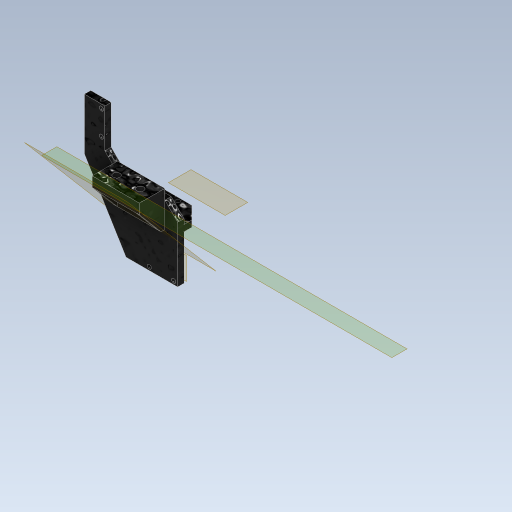
# Autodesk Inventor part: Suporte Switch Límite
Saved by Autodesk Inventor 2024.2 (Build 282272000, 272)
## iProperties
Created: 2024-01-17
Part Number: Suporte Switch Límite
Material: PET Plastic
Document SubType Name: Modeling
Designer: juanp
Density: 1.541 g/cm^3
Appearance: Black
Author: juanp
Autodesk Inventor part; units mm, degrees
ref_plane "YZ Plane" through (0, 0, 0) normal (1, 0, 0) x (0, 1, 0)
ref_plane "XZ Plane" through (0, 0, 0) normal (0, 1, 0) x (-1, 0, 0)
ref_plane "Work Plane1" through (0, 3, 3) normal (0, 0, 1) x (1, 0, 0)
sketch "Sketch1" plane through (0, 3, 3) normal (0, 0, 1) x (1, 0, 0)
  line L0 (-20.25, 5.05) -> (-20.25, -11.05) projected
  line L1 (-20.25, -11.05) -> (20.25, -11.05) projected
  line L2 (20.25, -11.05) -> (20.25, 5.05) projected
  line L3 (20.25, 5.05) -> (-20.25, 5.05) projected
  line L4 (-7.83, -4.67) -> (-7.83, -4.03) construction
  line L5 (-8.47, -4.67) -> (-7.83, -4.67) construction
  line L6 (-8.47, -4.03) -> (-8.47, -4.67) construction
  line L7 (-7.83, -4.03) -> (-8.47, -4.03) construction
  line L8 (-7.83, -7.17) -> (-7.83, -6.53) construction
  line L9 (-8.47, -7.17) -> (-7.83, -7.17) construction
  line L10 (-8.47, -6.53) -> (-8.47, -7.17) construction
  line L11 (-7.83, -6.53) -> (-8.47, -6.53) construction
  line L12 (2.725, -2.1031) -> (1.875, -2.1031) construction
  line L13 (2.725, -2.9531) -> (2.725, -2.1031) construction
  line L14 (1.875, -2.9531) -> (2.725, -2.9531) construction
  line L15 (1.875, -2.1031) -> (1.875, -2.9531) construction
  line L16 (7.875, -2.1031) -> (7.025, -2.1031) construction
  line L17 (7.875, -2.9531) -> (7.875, -2.1031) construction
  line L18 (7.025, -2.9531) -> (7.875, -2.9531) construction
  line L19 (7.025, -2.1031) -> (7.025, -2.9531) construction
  line L20 (13.025, -2.1031) -> (12.175, -2.1031) construction
  line L21 (13.025, -2.9531) -> (13.025, -2.1031) construction
  line L22 (12.175, -2.9531) -> (13.025, -2.9531) construction
  line L23 (12.175, -2.1031) -> (12.175, -2.9531) construction
  line L24 (-7.83, -2.17) -> (-7.83, -1.53) construction
  line L25 (-8.47, -2.17) -> (-7.83, -2.17) construction
  line L26 (-8.47, -1.53) -> (-8.47, -2.17) construction
  line L27 (-7.83, -1.53) -> (-8.47, -1.53) construction
  line L28 (-7.83, 0.33) -> (-7.83, 0.97) construction
  line L29 (-8.47, 0.33) -> (-7.83, 0.33) construction
  line L30 (-8.47, 0.97) -> (-8.47, 0.33) construction
  line L31 (-7.83, 0.97) -> (-8.47, 0.97) construction
  circle A0 centre (-16.75, 2.4) radius 1.5 construction
  circle A1 centre (17.15, -8.4) radius 1.5 construction
  circle A2 centre (-1.95, -8.4) radius 1.5 construction
  circle A3 centre (-16.75, -8.4) radius 1.5 construction
  line L32 (-53, 42.95) -> (-36.9, 42.95) projected
  line L33 (-36.9, 42.95) -> (-36.9, 83.45) projected
  line L34 (-36.9, 83.45) -> (-53, 83.45) projected
  line L35 (-53, 83.45) -> (-53, 42.95) projected
  line L36 (-43.28, 55.37) -> (-43.92, 55.37) construction
  line L37 (-43.28, 54.73) -> (-43.28, 55.37) construction
  line L38 (-43.92, 54.73) -> (-43.28, 54.73) construction
  line L39 (-43.92, 55.37) -> (-43.92, 54.73) construction
  line L40 (-40.78, 55.37) -> (-41.42, 55.37) construction
  line L41 (-40.78, 54.73) -> (-40.78, 55.37) construction
  line L42 (-41.42, 54.73) -> (-40.78, 54.73) construction
  line L43 (-41.42, 55.37) -> (-41.42, 54.73) construction
  line L44 (-45.8469, 65.925) -> (-45.8469, 65.075) construction
  line L45 (-44.9969, 65.925) -> (-45.8469, 65.925) construction
  line L46 (-44.9969, 65.075) -> (-44.9969, 65.925) construction
  line L47 (-45.8469, 65.075) -> (-44.9969, 65.075) construction
  line L48 (-45.8469, 71.075) -> (-45.8469, 70.225) construction
  line L49 (-44.9969, 71.075) -> (-45.8469, 71.075) construction
  line L50 (-44.9969, 70.225) -> (-44.9969, 71.075) construction
  line L51 (-45.8469, 70.225) -> (-44.9969, 70.225) construction
  line L52 (-45.8469, 76.225) -> (-45.8469, 75.375) construction
  line L53 (-44.9969, 76.225) -> (-45.8469, 76.225) construction
  line L54 (-44.9969, 75.375) -> (-44.9969, 76.225) construction
  line L55 (-45.8469, 75.375) -> (-44.9969, 75.375) construction
  line L56 (-45.78, 55.37) -> (-46.42, 55.37) construction
  line L57 (-45.78, 54.73) -> (-45.78, 55.37) construction
  line L58 (-46.42, 54.73) -> (-45.78, 54.73) construction
  line L59 (-46.42, 55.37) -> (-46.42, 54.73) construction
  line L60 (-48.28, 55.37) -> (-48.92, 55.37) construction
  line L61 (-48.28, 54.73) -> (-48.28, 55.37) construction
  line L62 (-48.92, 54.73) -> (-48.28, 54.73) construction
  line L63 (-48.92, 55.37) -> (-48.92, 54.73) construction
  circle A4 centre (-50.35, 46.45) radius 1.5 construction
  circle A5 centre (-39.55, 80.35) radius 1.5 construction
  circle A6 centre (-39.55, 61.25) radius 1.5 construction
  circle A7 centre (-39.55, 46.45) radius 1.5 construction
  circle A8 centre (-1.95, -8.4) radius 1.65
  circle A9 centre (17.15, -8.4) radius 1.65
  circle A10 centre (-39.55, 61.25) radius 1.65
  circle A11 centre (-39.55, 80.35) radius 1.65
  circle A12 centre (-1.95, -8.4) radius 2.65
  circle A13 centre (17.15, -8.4) radius 2.65
  circle A14 centre (-39.55, 61.25) radius 2.65
  circle A15 centre (-39.55, 80.35) radius 2.65
  line L64 (-20.25, 20.94) -> (20.25, 20.94) projected
  line L65 (-20.25, 20.94) -> (20.25, 20.94)
  line L66 (20.25, 20.94) -> (20.25, 28.94)
  line L67 (20.25, 28.94) -> (-20.25, 28.94)
  line L68 (-20.25, 28.94) -> (-20.25, 20.94)
  line L69 (-20.25, -11.05) -> (-53, 42.95)
  line L70 (20.25, 5.05) -> (20.25, 20.94)
  line L71 (20.25, 28.94) -> (20.25, 42.95)
  line L72 (20.25, 42.95) -> (-36.9, 42.95)
  line L73 (-25.9738, 88.007) -> (-9.8738, 88.007)
  line L74 (-9.8738, 88.007) -> (-9.8738, 47.507)
  line L75 (-9.8738, 47.507) -> (-25.9738, 47.507)
  line L76 (-25.9738, 47.507) -> (-25.9738, 88.007)
  line L77 (-12.5238, 84.907) -> (-12.5238, 65.807) construction
  circle A16 centre (-12.5238, 84.907) radius 1.5
  circle A17 centre (-12.5238, 65.807) radius 1.5
  point P0 (0, -3)
  dimension "d0" = 0.15
  dimension "d2" = 1
  dimension "d3" = 8
  dimension "d37" = 40.5
  dimension "d38" = 16.1
  dimension "d39" = 19.1
  dimension "d40" = 3
  dimension "d41" = 2.65
  dimension "d42" = 3.1
  dimension "d43" = 3
  dimension "d44" = 19.1
  dimension "d45" = 3.1
  dimension "d46" = 2.65
  dimension "d47" = 16.1
  dimension "d48" = 40.5
  constraints: 26 end point, 10 centre point, 7 equal radius, 4 parallel, 3 horizontal, 2 coincident, 2 perpendicular, 1 collinear, 1 point on line, 1 vertical
  measures "d0" radial gap between concentric circles of A2 A8
  measures "d2" radial gap between concentric circles of A12 A8
  measures "d3" distance between parallel lines of L67 L64
  measures "d37" distance of L32.end L33.end
  measures "d38" distance of L33.end L34.end
  measures "d39" distance of A5.centre A6.centre
  measures "d40" diameter of A5
  measures "d41" distance from line of L33 A5.centre
  measures "d42" distance from line of L34 A5.centre
  measures "d43" diameter of A16
  measures "d44" distance of L77.start L77.end
  measures "d45" distance from line of L73 L77.start
  measures "d46" distance between parallel lines of L74 L77
  measures "d47" distance of L73.start L73.end
  measures "d48" distance between parallel lines of L73 L75
extrude "Extrusion1" add sketch "Sketch1" along normal blind 5 contours A12 | A13 | L3 L2 L1 L0 | L0 L69 L32 L72 L71 L67 L68 L64 L70 L3 | A14 | A15 | L35 L34 L33 L32
sketch "Sketch2" plane through (0, 3, 8) normal (0, 0, 1) x (1, 0, 0)
  line L0 (20.25, 20.94) -> (-20.25, 20.94) projected
  line L1 (-20.25, 28.94) -> (20.25, 28.94) projected
  line L2 (-20.25, 20.94) -> (20.25, 20.94)
  line L3 (20.25, 20.94) -> (20.25, 28.94)
  line L4 (20.25, 28.94) -> (-20.25, 28.94)
  line L5 (-20.25, 28.94) -> (-20.25, 20.94)
  line L6 (-20.25, 20.94) -> (-20.25, 28.94) projected
  line L7 (-20.25, 23.94) -> (20.25, 23.94)
  point P0 (0, -3)
  dimension "d6" = 5
  constraints: 10 end point, 2 horizontal, 2 parallel, 2 point on line, 1 perpendicular
  measures "d6" distance between parallel lines of L1 L7
ref_plane "Work Plane2" through (-20.25, 19.44, -13.1) normal (0, 0, -1) x (0, 1, 0)
extrude "Extrusion2" add sketch "Sketch2" against normal up to surface (21.1 mm away) contours L7 L5 L1 L3
extrude "Extrusion3" add sketch "Sketch2" against normal up to surface (5 mm away) contours L0 L5 L7 L3
ref_plane "Work Plane3" through (0, 23.94, -36.1658) normal (0, 1, 0) x (-1, 0, 0)
sketch "Sketch3" plane through (0, 23.94, -36.1658) normal (0, 1, 0) x (-1, 0, 0)
  line L0 (-20.25, 39.1658) -> (-20.25, 23.0658) construction
  line L1 (-20.25, 23.0658) -> (20.25, 23.0658) construction
  line L2 (20.25, 23.0658) -> (20.25, 39.1658) construction
  line L3 (20.25, 39.1658) -> (-20.25, 39.1658) construction
  line L4 (-7.83, 29.4458) -> (-7.83, 30.0858) construction
  line L5 (-8.47, 29.4458) -> (-7.83, 29.4458) construction
  line L6 (-8.47, 30.0858) -> (-8.47, 29.4458) construction
  line L7 (-7.83, 30.0858) -> (-8.47, 30.0858) construction
  line L8 (-7.83, 26.9458) -> (-7.83, 27.5858) construction
  line L9 (-8.47, 26.9458) -> (-7.83, 26.9458) construction
  line L10 (-8.47, 27.5858) -> (-8.47, 26.9458) construction
  line L11 (-7.83, 27.5858) -> (-8.47, 27.5858) construction
  line L12 (2.725, 32.0128) -> (1.875, 32.0128) construction
  line L13 (2.725, 31.1628) -> (2.725, 32.0128) construction
  line L14 (1.875, 31.1628) -> (2.725, 31.1628) construction
  line L15 (1.875, 32.0128) -> (1.875, 31.1628) construction
  line L16 (7.875, 32.0128) -> (7.025, 32.0128) construction
  line L17 (7.875, 31.1628) -> (7.875, 32.0128) construction
  line L18 (7.025, 31.1628) -> (7.875, 31.1628) construction
  line L19 (7.025, 32.0128) -> (7.025, 31.1628) construction
  line L20 (13.025, 32.0128) -> (12.175, 32.0128) construction
  line L21 (13.025, 31.1628) -> (13.025, 32.0128) construction
  line L22 (12.175, 31.1628) -> (13.025, 31.1628) construction
  line L23 (12.175, 32.0128) -> (12.175, 31.1628) construction
  line L24 (-7.83, 31.9458) -> (-7.83, 32.5858) construction
  line L25 (-8.47, 31.9458) -> (-7.83, 31.9458) construction
  line L26 (-8.47, 32.5858) -> (-8.47, 31.9458) construction
  line L27 (-7.83, 32.5858) -> (-8.47, 32.5858) construction
  line L28 (-7.83, 34.4458) -> (-7.83, 35.0858) construction
  line L29 (-8.47, 34.4458) -> (-7.83, 34.4458) construction
  line L30 (-8.47, 35.0858) -> (-8.47, 34.4458) construction
  line L31 (-7.83, 35.0858) -> (-8.47, 35.0858) construction
  circle A0 centre (-16.75, 36.5158) radius 1.5 construction
  circle A1 centre (17.15, 25.7158) radius 1.5 construction
  circle A2 centre (-1.95, 25.7158) radius 1.5 construction
  circle A3 centre (-16.75, 25.7158) radius 1.5 construction
  circle A4 centre (-1.95, 25.7158) radius 1.65
  circle A5 centre (-16.75, 25.7158) radius 1.65 construction
  circle A6 centre (17.15, 25.7158) radius 1.65
  point P0 (0, 36.1658)
  dimension "d11" = 0.15
  dimension "d12" = 0.15
  constraints: 3 centre point, 1 equal radius
  measures "d11" radial gap between concentric circles of A2 A4
  measures "d12" radial gap between concentric circles of A3 A5
extrude "Extrusion4" cut sketch "Sketch3" along normal through all
chamfer "Chamfer1" distance 10 angle 45 3 edges at (-36.9, 45.95, 5.5) (20.25, 45.95, 5.5) (20.25, 29.44, -13.1)
ref_plane "Work Plane4" through (451.95, 53.95, 22.59) normal (0, -1, 0) x (0, 0, -1)
sketch "Sketch4" plane through (451.95, 53.95, 22.59) normal (0, -1, 0) x (0, 0, -1)
  line L0 (9.16, -250) -> (14.08, -250) construction
  line L1 (9.16, -500) -> (9.16, -250) construction
  line L2 (14.08, -500) -> (9.16, -500) construction
  line L3 (14.08, -500) -> (14.08, -250) construction
  line L4 (-10.84, -250) -> (0, -250) construction
  line L5 (-10.84, -500) -> (-10.84, -250) construction
  line L6 (0, -500) -> (-10.84, -500) construction
  line L7 (0, -500) -> (0, -250) construction
  line L8 (14.58, -478.85) -> (-5.42, -478.85)
  line L9 (-5.42, -478.85) -> (-5.42, -441.7)
  line L10 (-5.42, -441.7) -> (14.58, -441.7)
  line L11 (14.58, -441.7) -> (14.58, -478.85)
  line L12 (9.16, -480.6966) -> (0, -480.6966) construction
  line L13 (4.58, -478.85) -> (4.58, -441.7) construction
  line L14 (4.58, -478.85) -> (4.58, -460.275) construction
  line L15 (4.58, -460.275) -> (4.58, -441.7) construction
  circle A0 centre (4.58, -469.5625) radius 2.65
  circle A1 centre (4.58, -450.9875) radius 2.65
  point P0 (22.59, -451.95)
  point P1 (4.58, -480.6966)
  point P2 (-5.42, -460.275)
  point P3 (14.59, -441.7)
  point P4 (14.59, -478.85)
  dimension "d18" = 20
  dimension "d19" = 5.3
  constraints: 16 end point, 7 midpoint, 5 point on line, 2 centre point, 2 parallel, 2 perpendicular, 1 collinear, 1 equal radius, 1 horizontal
  measures "d18" distance from line of point (-5.42, -460.275) L11
  measures "d19" diameter of A1
sketch "Sketch5" plane through (0, 3, 8) normal (0, 0, 1) x (1, 0, 0)
  line L0 (-26.9, 50.95) -> (10.25, 50.95) projected
  line L1 (-26.9, 22.95) -> (10.25, 22.95)
  line L2 (10.25, 22.95) -> (10.25, 42.95)
  line L3 (10.25, 42.95) -> (-26.9, 42.95)
  line L4 (-26.9, 42.95) -> (-26.9, 22.95)
  line L5 (-26.9, 32.95) -> (-8.325, 32.95) construction
  line L6 (-8.325, 32.95) -> (10.25, 32.95) construction
  circle A0 centre (-17.6125, 32.95) radius 2.65
  circle A1 centre (0.9625, 32.95) radius 2.65
  point P0 (0, -3)
  dimension "d20" = 20
  dimension "d21" = 5.3
  dimension "d22" = 5.3
  constraints: 12 end point, 4 midpoint, 2 centre point, 2 coincident, 2 horizontal, 2 parallel, 1 collinear, 1 perpendicular
  measures "d20" distance between parallel lines of L3 L1
  measures "d21" diameter of A0
  measures "d22" diameter of A1
extrude "Extrusion5" add sketch "Sketch4" along normal up to surface (8 mm away) separate body
extrude "Extrusion6" add sketch "Sketch5" along normal blind 3 bodies 2
ref_plane "Work Plane5" through (-26.9, 25.95, 11) normal (0, -0.6478695, 0.7617513) x (1, 0, 0)
sketch "Sketch6" plane through (-26.9, 25.95, 11) normal (0, -0.6478695, 0.7617513) x (1, 0, 0)
  line L0 (0, 0) -> (37.15, 0) projected
  line L1 (37.15, 26.2553) -> (0, 26.2553) projected
  line L2 (0, 0) -> (3, 0)
  line L3 (3, 0) -> (3, 26.2553)
  line L4 (3, 26.2553) -> (0, 26.2553)
  line L5 (0, 26.2553) -> (0, 0)
  line L6 (37.15, 0) -> (34.15, 0)
  line L7 (34.15, 0) -> (34.15, 26.2553)
  line L8 (34.15, 26.2553) -> (37.15, 26.2553)
  line L9 (37.15, 26.2553) -> (37.15, 0)
  point P0 (26.9, -26.894)
  point P1 (0, 26.2553)
  point P2 (3, 0)
  point P3 (37.15, 26.2553)
  point P4 (34.15, 0)
  dimension "d31" = 3
  dimension "d32" = 3
  constraints: 16 end point, 4 parallel, 2 horizontal, 2 perpendicular, 2 point on line
  measures "d31" distance between parallel lines of L7 L9
  measures "d32" distance between parallel lines of L5 L3
extrude "Extrusion7" add sketch "Sketch6" against normal up to next contours L5 L1 L3 L0 | L7 L1 L9 L0 bodies 2
sketch "Sketch7" plane through (0, 3, 11) normal (0, 0, 1) x (1, 0, 0)
  circle A0 centre (0.9625, 32.95) radius 2.65 projected
  circle A1 centre (-17.6125, 32.95) radius 2.65 projected
  line L0 (-23.9, 42.95) -> (-23.9, 22.95) projected
  line L1 (-23.9, 22.95) -> (7.25, 22.95) projected
  line L2 (7.25, 22.95) -> (7.25, 42.95) projected
  line L3 (-23.9, 42.95) -> (7.25, 42.95) projected
  point P0 (0, -3)
extrude "Extrusion8" cut sketch "Sketch7" against normal through all contours A0 | A1 bodies 2 1
body "Solid1"
body "Solid2"
